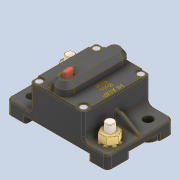
# Autodesk Inventor part: COTS_am-0282_MainBreaker
Saved by Autodesk Inventor 2021 (Build 250183000, 183)
## iProperties
Created: 2015-01-22
Part Number: COTS_am-0282_MainBreaker
Material: Main Breaker Material
Description: STEP AP214
Document SubType Name: Modeling
Designer: Marshall
Mass: 109.97 g
Surface Area: 68.1755 cm^2
Volume: 34.547 cm^3
Density: 3.18319 g/cm^3
Appearance: Default(1)
Sending System: SolidWorks 2014
Preprocessor: SwSTEP 2.0
Title: am-0282 120a Circuit Breaker.STEP
Revision Number: ANY
Autodesk Inventor part; units mm, degrees
ref_plane "YZ Plane" through (0, 0, 0) normal (1, 0, 0) x (0, 1, 0)
ref_plane "XZ Plane" through (0, 0, 0) normal (0, 1, 0) x (-1, 0, 0)
ref_plane "XY Plane" through (0, 0, 0) normal (0, 0, 1) x (1, 0, 0)
surface "Composite1"
sketch "Sketch1" plane through (-24.384, 0, 24.13) normal (0, -1, 0) x (1, 0, 0)
  line L0 (42.291, -48.26) -> (6.477, -48.26) projected
  line L1 (42.291, 0) -> (6.477, 0)
  line L2 (6.477, 0) -> (6.477, -48.26)
  line L3 (6.477, -48.26) -> (42.291, -48.26)
  line L4 (42.291, -48.26) -> (42.291, 0) construction
  line L5 (42.291, 0) -> (6.477, -48.26) construction
  line L6 (6.477, 0) -> (42.291, -48.26) construction
  line L7 (42.281, -0.01) -> (6.487, -0.01)
  line L8 (6.487, -0.01) -> (6.487, -48.25)
  line L9 (6.487, -48.25) -> (42.281, -48.25)
  line L10 (42.281, -48.25) -> (42.281, -0.01)
  point P0 (24.384, -24.13)
  dimension "d2" = 0.01
  constraints: 20 end point, 4 parallel, 2 midpoint, 2 perpendicular, 1 horizontal, 3 other
  measures "d2" distance between parallel lines of L4 L10
extrude "Extrusion1" add sketch "Sketch1" against normal blind 20
sketch "Sketch2" plane through (-24.384, 0, 24.13) normal (0, -1, 0) x (1, 0, 0)
  point P0 (24.384, -24.13)
sketch "Sketch3" plane through (-24.384, 0, 24.13) normal (0, -1, 0) x (1, 0, 0)
  line L0 (6.487, -0.01) -> (6.487, -48.25) projected
  line L1 (6.487, -48.25) -> (42.281, -48.25) projected
  line L2 (42.281, -48.25) -> (42.281, -0.01) projected
  line L3 (42.281, -0.01) -> (6.487, -0.01) projected
  point P0 (24.384, -24.13)
extrude "Extrusion2" cut sketch "Sketch3" against normal blind 0.01
body "Solid1"
body "Srf1"
